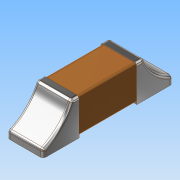
# Autodesk Inventor part: GRM155R61E105KA12D Capacitor
Saved by Autodesk Inventor 2016 (Build 200138000, 138)
## iProperties
Created: 2019-08-18
Part Number: GRM155R61E105KA12D Capacitor
Material: Laminate, Ivory, Matte
Document SubType Name: Modeling
Designer: Orest
Mass: 0.000451825 g
Surface Area: 0.0333144 cm^2
Volume: 0.000327409 cm^3
Density: 1.38 g/cm^3
Appearance: Smooth - Ivory(2)
Author: Orest
Autodesk Inventor part; units mm, degrees
ref_plane "YZ Plane" through (0, 0, 0) normal (1, 0, 0) x (0, 1, 0)
ref_plane "XZ Plane" through (0, 0, 0) normal (0, 1, 0) x (-1, 0, 0)
ref_plane "XY Plane" through (0, 0, 0) normal (0, 0, 1) x (1, 0, 0)
sketch "Sketch10" plane through (0, 0, 0) normal (0, 0, 1) x (1, 0, 0)
  line L0 (-0.4, 0.2375) -> (0.4, 0.2375)
  line L1 (0.4, 0.2375) -> (0.4, -0.2375)
  line L2 (0.4, -0.2375) -> (-0.4, -0.2375)
  line L3 (-0.4, -0.2375) -> (-0.4, 0.2375)
  point P0 (0, 0)
  point P1 (-0.4, 0)
  point P2 (0, 0.2375)
  dimension "d7" = 0.8
  dimension "d8" = 0.475
  constraints: 8 end point, 2 midpoint, 2 parallel, 1 horizontal, 1 horizontal alignment, 1 perpendicular, 1 vertical alignment
  measures "d7" distance of L1.end L2.end
  measures "d8" distance of L0.end L1.end
extrude "Extrusion4" add sketch "Sketch10" along normal mid plane 0.475
sketch "Sketch11" plane through (0.4, -0.2375, 0.2375) normal (1, 0, 0) x (0, 0, -1)
  line L0 (0, 0.475) -> (0.475, 0.475) construction
  line L1 (0, 0) -> (0, 0.475) construction
  line L2 (0, 0) -> (0.475, 0) construction
  line L3 (0.475, 0.475) -> (0.475, 0) construction
  line L4 (0.4875, 0.4875) -> (-0.0125, 0.4875)
  line L5 (-0.0125, 0.4875) -> (-0.0125, -0.0125)
  line L6 (-0.0125, -0.0125) -> (0.4875, -0.0125)
  line L7 (0.4875, -0.0125) -> (0.4875, 0.4875)
  line L8 (-0.0125, -0.0125) -> (0.4875, -0.0125)
  line L9 (0.4875, -0.0125) -> (0.4875, 0.0875)
  line L10 (0.4875, 0.0875) -> (-0.0125, 0.0875)
  line L11 (-0.0125, 0.0875) -> (-0.0125, -0.0125)
  point P0 (0.2375, 0.2375)
  dimension "d11" = 0.5
  dimension "d14" = 0.1
  constraints: 16 end point, 2 parallel, 1 horizontal, 1 perpendicular, 1 point on line, 3 other
  measures "d11" distance of L4.start L4.end
  measures "d14" distance between parallel lines of L6 L10
extrude "Extrusion5" add sketch "Sketch11" along normal blind 0.1
extrude "Extrusion6" add sketch "Sketch11" along normal blind 0.5 contours L7 L6 L5 L10
fillet "Fillet1" radius 0.75 1 edges at (0.5, -0.15, 0)
fillet "Fillet2" radius 0.0425 8 edges at (0.45, 0.25, -0.25) (0.45, 0.25, 0.25) (0.6608, 0.0108, 0.25) (0.6608, 0.0108, -0.25) (0.9, -0.2, -0.25) (0.9, -0.15, 0) (0.9, -0.2, 0.25) (0.5, 0.25, 0)
mirror "Mirror1" about plane through (0, 0, 0) normal (1, 0, 0) of "Extrusion5", "Fillet1", "Fillet2", "Extrusion6"
fillet "Fillet3" radius 0.03 4 edges at (0, 0.2375, -0.2375) (0, 0.2375, 0.2375) (0, -0.2375, -0.2375) (0, -0.2375, 0.2375)
equation "\"d9\" = d8"
body "Solid4"
